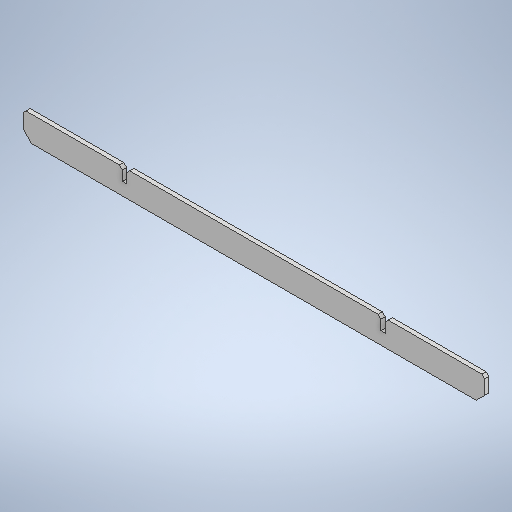
# Autodesk Inventor part: foot support
Saved by Autodesk Inventor 2025.2 (Build 292293000, 293)
## iProperties
Created: 2025-05-20
Part Number: foot support
Material: Generic
Document SubType Name: Sheet Metal
Designer: Caspe
Density: 1 g/cm^3
Sheet Metal Rule: Default_mm
Appearance: Default
Author: Caspe
Autodesk Inventor part; units mm, degrees
ref_plane "YZ Plane" through (0, 0, 0) normal (1, 0, 0) x (0, 1, 0)
ref_plane "XZ Plane" through (0, 0, 0) normal (0, 1, 0) x (-1, 0, 0)
ref_plane "XY Plane" through (0, 0, 0) normal (0, 0, 1) x (1, 0, 0)
sketch "Sketch1" plane through (0, 0, 0) normal (0, 0, 1) x (1, 0, 0)
  line L0 (0, 0) -> (327, 0)
  line L1 (327, 0) -> (327, 18)
  line L2 (327, 18) -> (0, 18)
  line L3 (0, 18) -> (0, 0)
  line L4 (163.5, 18) -> (163.5, 0)
  line L5 (73.5, 18) -> (70.3, 18)
  line L6 (70.3, 18) -> (70.3, 9)
  line L7 (70.3, 9) -> (73.5, 9)
  line L8 (73.5, 9) -> (73.5, 18)
  line L9 (256.7, 18) -> (256.7, 9)
  line L10 (256.7, 9) -> (253.5, 9)
  line L11 (253.5, 9) -> (253.5, 18)
  dimension "d0" = 327
  dimension "d1" = 18
  dimension "d2" = 3.2
  dimension "d3" = 9
  dimension "d4" = 180
  measures "d0" distance of L2.end L1.end
  measures "d1" distance of L1.end L0.end
  measures "d2" distance of L7.end L6.end
  measures "d3" distance of L6.end L5.end
  measures "d4" diameter of L8 L4
extrude "Plate1" add sketch "Sketch1" along normal blind 3 contours L3 L2 L6 L7 L8 L4 L0 | L4 L2 L11 L10 L9 L1 L0
chamfer "Corner Chamfer1" distance 6 angle 45 2 edges at (0, 0, 1.5) (327, 0, 1.5)
chamfer "Corner Chamfer2" distance 2 angle 45 6 edges at (327, 18, 1.5) (256.7, 18, 1.5) (253.5, 18, 1.5) (73.5, 18, 1.5) (70.3, 18, 1.5) (0, 18, 1.5)
equation "\"d5\" = Thickness"
equation "\"BendRadius\" = Thickness"
equation "\"BendReliefWidth\" = Thickness"
equation "\"BendReliefDepth\" = 0.5 * Thickness"
equation "\"CornerReliefSize\" = 4 * Thickness"
equation "\"MinimumRemnant\" = 2 * Thickness"
equation "\"TransitionRadius\" = BendRadius"
equation "\"JacobiRadiusSize\" = BendRadius"
equation "\"GapSize\" = Thickness"
equation "\"Thickness\" = 3"
body "Solid1"
